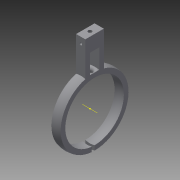
# Autodesk Inventor part: valvula-cocacola-v1
Saved by Autodesk Inventor 2015 SP1 (Build 190203100, 203)
## iProperties
Created: 2015-07-03
Part Number: valvula-cocacola-v1
Material: Genérico
Document SubType Name: Modeling
Designer: Javier
Density: 1 g/cm^3
Appearance: Valor por defecto
Author: Javier
Autodesk Inventor part; units mm, degrees
ref_plane "YZ Plane" through (0, 0, 0) normal (1, 0, 0) x (0, 1, 0)
ref_plane "XZ Plane" through (0, 0, 0) normal (0, 1, 0) x (-1, 0, 0)
ref_plane "XY Plane" through (0, 0, 0) normal (0, 0, 1) x (1, 0, 0)
sketch "Boceto1" plane through (0, 0, 0) normal (0, 0, 1) x (1, 0, 0)
  point P0 (0, 0)
sketch "Boceto2" plane through (0, 0, 0) normal (0, 1, 0) x (-1, 0, 0)
  line L0 (0, 0) -> (0, -32.5)
  arc A0 (-5, -31.7) -> (5, -31.7) centre (0, -16.475) ccw
  line L1 (5, -31.7) -> (-5, -31.7) construction
  line L2 (5, -31.7) -> (15, -31.7) construction
  line L3 (5, -31.7) -> (5, -36.7)
  line L4 (-5, -31.7) -> (-5, -36.7)
  arc A1 (-5, -36.7) -> (5, -36.7) centre (0, -18.7402) ccw
  line L5 (19, 0) -> (-9, 0) projected
  dimension "d0" = 32.5
  dimension "d1" = 10
  dimension "d2" = 180
  dimension "d3" = 5
  constraints: 10 end point, 5 point on circle, 2 centre point, 2 vertical, 1 collinear, 1 horizontal, 1 perpendicular
  measures "d0" distance of L0.start L0.end
  measures "d1" distance of L1.start L1.end
  measures "d2" angle of L1 L2
  measures "d3" distance of L1.start L3.end
revolve "Revolución1" add sketch "Boceto2" angle 355 about axis through (-10, 0, 0) along (1, 0, 0)
sketch "Boceto3" plane through (-5, 0, -36.7) normal (-1, 0, 0) x (0, 0, 1)
  arc A0 (5.1206, -2.7628) -> (5, 0) centre (36.7, 0) ccw projected
  arc A1 (-0.5408, -3.2581) -> (-0.683, 0) centre (36.7, 0) ccw projected
  arc A2 (5.1206, -2.7628) -> (5, 0) centre (36.7, 0) ccw projected
  line L0 (36.7, 0) -> (124.9794, 0)
  arc A3 (4.3237, -2.8326) -> (4.2, 0) centre (36.7, 0) ccw projected
  line L1 (69.2, 0) -> (69.2, -10)
  line L2 (69.2, -10) -> (109.2, -10)
  line L3 (109.2, -10) -> (109.2, 10)
  line L4 (109.2, 10) -> (69.2, 10)
  line L5 (69.2, 10) -> (69.2, 0)
  line L6 (94.2, -5) -> (69.2, -5)
  line L7 (94.2, 5) -> (69.2, 5)
  line L8 (94.2, -5) -> (94.2, 5)
  dimension "d11" = 10
  dimension "d12" = 40
  dimension "d13" = 20
  dimension "d14" = 90
  dimension "d28" = 25
  dimension "d29" = 25
  constraints: 18 end point, 3 perpendicular, 2 midpoint, 2 point on line, 1 horizontal, 1 point on circle, 1 tangent
  measures "d11" distance of L1.start L1.end
  measures "d12" distance of L1.end L2.end
  measures "d13" distance of L2.end L3.end
  measures "d14" angle of L4 L3
  measures "d28" distance of L6.start L6.end
  measures "d29" distance of L7.start L7.end
extrude "Extrusión1" add sketch "Boceto3" against normal blind 10 contours L2 L1 L6 A1 | A1 L6 L8 L0 L3 L2 | L0 L8 L7 A1 L4 L3 | L7 L5 L4 A1
sketch "Boceto4" plane through (-5, -10, 72.5) normal (0, 0, 1) x (1, 0, 0)
  line L0 (0, 0) -> (0, 20) projected
  line L1 (0, 0) -> (10, 0) projected
  line L2 (10, 20) -> (10, 0) projected
  line L3 (0, 20) -> (10, 20) projected
  circle A0 centre (5, 10) radius 2
  point P0 (5, 10)
  dimension "d17" = 4
  constraints: 1 centre point, 1 coincident
  measures "d17" diameter of A0
extrude "Extrusión2" cut sketch "Boceto4" against normal up to surface (15 mm away) contours A0
sketch "Boceto5" plane through (-5, -5, 57.5) normal (0, 0, -1) x (-1, 0, 0)
  circle A0 centre (-5, 5) radius 2 projected
  line L0 (0, -5) -> (0, 15) projected
  line L1 (0, -5) -> (-10, -5) projected
  line L2 (-10, 15) -> (-10, -5) projected
  line L3 (0, 15) -> (-10, 15) projected
  circle A1 centre (-5, 5) radius 2 projected
  circle A2 centre (-5, 5) radius 2 projected
  circle A3 centre (-5, 5) radius 2 projected
  circle A4 centre (-5, 5) radius 2.5
  point P0 (-5, 5)
  dimension "d20" = 5
  constraints: 1 centre point, 1 coincident
  measures "d20" diameter of A4
extrude "Extrusión3" cut sketch "Boceto5" along normal blind 40 contours A0 | A4
fillet "Empalme1" radius 3 2 edges at (-2.4099, 0.6651, 37.2207) (2.4098, -0.6655, 37.2207)
